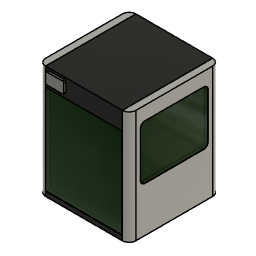
H2D concept v1 (Autodesk Fusion 360 design; units mm, degrees)
Autodesk Fusion 360 part; units mm, degrees
note: some values were not read from the file. Chosen so that the rebuilt part matches the saved one: which bodies a step acts on.
sketch "Sketch1" plane through (0, 0, 0) normal (0, 0, 1) x (1, 0, 0)
  line L0 (0, 0) -> (40, 0)
  line L1 (40, 0) -> (40, 40)
  line L2 (40, 40) -> (0, 40)
  line L3 (0, 40) -> (0, 0)
  constraint horizontal L0
  constraint vertical L1
  constraint horizontal L2
  constraint vertical L3
  constraint coincident L0.start L3.end
extrude "Extrude1" add sketch "Sketch1" along normal blind 50 makes body 1
fillet "Fillet1" radius 3 4 edges at (0, 0, 25) (40, 0, 25) (40, 40, 25) (0, 40, 25) on bodies 1
sketch "Sketch2" plane through (0, 0, 0) normal (0, -1, 0) x (1, 0, 0)
  line L0 (37, 0) -> (37, 50)
  line L1 (37, 50) -> (3, 50)
  line L2 (3, 50) -> (3, 0)
  line L3 (3, 0) -> (37, 0)
  line L4 (37, 2) -> (3, 2)
  line L5 (3, 2) -> (3, 42)
  line L6 (3, 42) -> (37, 42)
  line L7 (37, 42) -> (37, 2)
  constraint horizontal L4
  constraint vertical L5
  constraint horizontal L6
  constraint vertical L7
  constraint coincident L2 L5.end
  constraint coincident L0 L4.start
extrude "Extrude2" cut sketch "Sketch2" against normal blind 2 contours L0 L2 L4 L5 L6 L7 bodies 1
extrude "Extrude3" add 1 faces at (14.3333, 2, 28.6667) along direction (0, -1, 0) blind 2 separate body on bodies 1 makes body 2
scale "Scale1" factor 0.995 about (3, 0, 42) bodies 2
split "Split1" by plane through (3, 1.99, 42) normal (-1, 0, 0) bodies 1 makes body 3 at (0, 25.6667, 16.6667)
split "Split2" by plane through (37, 0, 2) normal (-1, 0, 0) bodies 1 makes body 4 at (3, 27.3333, 30.6667)
sketch "Sketch3" plane through (40, 0, 0) normal (1, 0, 0) x (0, 1, 0)
  line L0 (37, 0) -> (37, 50)
  line L1 (37, 50) -> (3, 50)
  line L2 (3, 50) -> (3, 0)
  line L3 (3, 0) -> (37, 0)
  line L4 (5, 44) -> (35, 44)
  line L5 (35, 44) -> (35, 20)
  line L6 (35, 20) -> (5, 20)
  line L7 (5, 20) -> (5, 44)
  circle A0 centre (7, 42) radius 2
  circle A1 centre (33, 42) radius 2
  circle A2 centre (33, 22) radius 2
  circle A3 centre (7, 22) radius 2
  constraint horizontal L4
  constraint vertical L5
  constraint horizontal L6
  constraint vertical L7
  constraint tangent L4 A0
  constraint tangent L4 A1
  constraint tangent L5 A2
  constraint tangent L6 A3
extrude "Extrude4" cut sketch "Sketch3" against normal blind 1.5 contours L4 L5 L6 L7 A0 A1 A2 A3 | A0 | A1 | A3 | A2 bodies 1
extrude "Extrude5" add 1 faces at (38.5, 15.6667, 36) along direction (1, 0, 0) blind 1.5 separate body on bodies 1 makes body 5
scale "Scale2" factor 0.993 about (40, 7, 44) bodies 5
sketch "Sketch4" plane through (0, 0, 0) normal (0, -1, 0) x (1, 0, 0)
  line L0 (3, 42) -> (37, 42)
  line L1 (37, 42) -> (37, 50)
  line L2 (37, 50) -> (3, 50)
  line L3 (3, 50) -> (3, 42)
  line L4 (4, 49) -> (12, 49)
  line L5 (12, 49) -> (12, 44)
  line L6 (12, 44) -> (4, 44)
  line L7 (4, 44) -> (4, 49)
  constraint horizontal L4
  constraint vertical L5
  constraint horizontal L6
  constraint vertical L7
extrude "Extrude6" add sketch "Sketch4" along normal blind 1.5 separate body contours L4 L5 L6 L7 makes body 6
fillet "Fillet2" radius 0.5 4 edges at (12, -0.75, 49) (12, -0.75, 44) (4, -0.75, 49) (4, -0.75, 44) on bodies 6
extrude "Extrude7" cut 1 faces at (9.1667, -1.5, 45.6667) along direction (0, 1, 0) blind 0.5 on bodies 6 bodies 6
